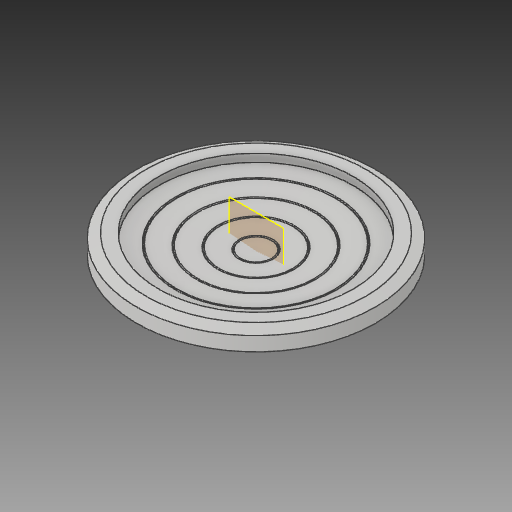
# Autodesk Inventor part: Caps 8mm Square Rounded Caps Male
Saved by Autodesk Inventor 2018 (Build 220112000, 112)
## iProperties
Created: 2017-12-12
Part Number: Caps 8mm Square Rounded Caps Male
Material: Generic
Document SubType Name: Modeling
Designer: Rus
Density: 1 g/cm^3
Appearance: Default
Author: Rus
Autodesk Inventor part; units mm, degrees
ref_plane "YZ Plane" through (0, 0, 0) normal (1, 0, 0) x (0, 1, 0)
ref_plane "XZ Plane" through (0, 0, 0) normal (0, 1, 0) x (-1, 0, 0)
ref_plane "XY Plane" through (0, 0, 0) normal (0, 0, 1) x (1, 0, 0)
sketch "Sketch1" plane through (0, 0, 0) normal (0, 1, 0) x (-1, 0, 0)
  circle A0 centre (0, 0) radius 4
  line L0 (0, 0) -> (4, 0) construction
  line L1 (0, 0) -> (0, -4) construction
  line L2 (0, 0) -> (-4, 0) construction
  line L3 (0, 0) -> (0, 4) construction
  dimension "d0" = 8
  constraints: 8 end point, 4 point on circle, 2 point on line, 1 centre point, 1 coincident, 1 horizontal, 1 perpendicular
  measures "d0" diameter of A0
extrude "Extrusion1" add sketch "Sketch1" against normal blind 3.5
ref_plane "Work Plane1" through (0, 0, 0) normal (0, 0, 1) x (1, 0, 0)
sketch "Sketch2" plane through (0, 0, 0) normal (0, 0, 1) x (1, 0, 0)
  line L0 (-4, 0) -> (4, 0) projected
  line L1 (4, 0) -> (12, 0)
  line L2 (19.05, 0.75) -> (19.05, 3)
  line L3 (17.55, 3.75) -> (15.55, 3.75)
  line L4 (0, 0) -> (0, 1.25)
  line L5 (4, 0) -> (4, 1.5959) construction
  line L6 (19.05, 0.75) -> (12, 0.75)
  line L7 (12, 0.75) -> (12, 0)
  line L8 (19.05, 3) -> (17.55, 3.75)
  line L9 (15.55, 2.5) -> (15.55, 3.75)
  line L10 (9.2263, 1.9917) -> (9.3609, 1.8771)
  line L11 (9.3609, 1.8771) -> (9.4755, 2.0117)
  line L12 (6.1006, 1.7404) -> (5.986, 1.6058)
  line L13 (5.986, 1.6058) -> (5.8514, 1.7204)
  line L14 (2.4765, 1.4491) -> (2.6111, 1.3345)
  line L15 (2.6111, 1.3345) -> (2.7257, 1.4691)
  line L16 (0, 1.25) -> (2.4765, 1.4491)
  line L17 (2.7257, 1.4691) -> (5.8514, 1.7204)
  line L18 (6.1006, 1.7404) -> (9.2263, 1.9917)
  line L19 (5.986, 1.6058) -> (5.986, 3.125) construction
  line L20 (9.3609, 1.8771) -> (9.3609, 3.125) construction
  line L21 (9.3609, 3.125) -> (5.986, 3.125) construction
  line L22 (5.986, 3.125) -> (2.6111, 3.125) construction
  line L23 (2.6111, 3.125) -> (0, 3.125) construction
  line L24 (2.4765, 1.4491) -> (2.7257, 1.4691) construction
  line L25 (5.8514, 1.7204) -> (6.1006, 1.7404) construction
  line L26 (9.2263, 1.9917) -> (9.4755, 2.0117) construction
  line L27 (2.6011, 1.4591) -> (2.6111, 1.3345) construction
  line L28 (5.986, 1.7312) -> (5.986, 1.6058) construction
  line L29 (2.6111, 1.3345) -> (2.6111, 3.125) construction
  line L30 (12.6012, 2.263) -> (12.7358, 2.1484)
  line L31 (12.7358, 2.1484) -> (12.8504, 2.283)
  line L32 (12.7358, 2.1484) -> (12.7358, 3.125) construction
  line L33 (9.4755, 2.0117) -> (12.6012, 2.263)
  line L34 (12.8504, 2.283) -> (15.55, 2.5)
  line L35 (9.3609, 3.125) -> (12.7358, 3.125) construction
  line L36 (12.7358, 3.125) -> (15.55, 3.125) construction
  point P0 (9.3609, 2.0025)
  dimension "d11" = 12
  dimension "d12" = 0.75
  dimension "d13" = 3
  dimension "d14" = 0.75
  dimension "d15" = 1.5
  dimension "d16" = 1.25
  dimension "d19" = 3.5
  dimension "d23" = 1.25
  dimension "d25" = 0.125
  dimension "d30" = 19.05
  constraints: 72 end point, 14 collinear, 11 perpendicular, 9 equal length, 6 point on line, 5 vertical, 3 horizontal, 2 midpoint
  measures "d11" distance between parallel lines of L7 L4
  measures "d12" distance of L6.end L1.end
  measures "d13" distance between parallel lines of L3 L6
  measures "d14" distance from line of L2.end L3
  measures "d15" distance from line of L2 L3.start
  measures "d16" distance of L4.start L4.end
  measures "d19" horizontal distance of L3.end L2.end
  measures "d23" vertical distance of L4.end L9.start
  measures "d25" distance of L27.start L14.end
  measures "d30" distance between parallel lines of L2 L4
revolve "Revolution1" add sketch "Sketch2" angle 360 about axis through (0, 0, 0) along (0, 1, 0)
sketch "Sketch3" plane through (0, -3.5, 0) normal (0, -1, 0) x (1, 0, 0)
  circle A0 centre (0, 0) radius 5.986 projected
  arc A1 (0, 5.986) -> (0, -5.986) centre (0, 0) ccw
  line L0 (0, -5.986) -> (0, 5.986)
  constraints: 4 point on circle, 2 end point, 1 centre point, 1 coincident, 1 line through centre, 1 vertical, 1 vertical alignment
extrude "Extrusion2" add sketch "Sketch3" along normal blind 2 contours L0 A0 picked at (-2.1196, -1.0755)
body "Solid1"
